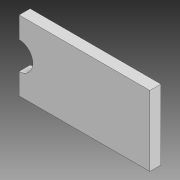
# Autodesk Inventor part: LED Backing
Saved by Autodesk Inventor 2020 (Build 240168000, 168)
## iProperties
Created: 2020-08-04
Part Number: LED Backing
Material: Generic
Document SubType Name: Modeling
Designer: DDeGo
Density: 1 g/cm^3
Appearance: Default
Author: DDeGo
Autodesk Inventor part; units mm, degrees
ref_plane "YZ Plane" through (0, 0, 0) normal (1, 0, 0) x (0, 1, 0)
ref_plane "XZ Plane" through (0, 0, 0) normal (0, 1, 0) x (-1, 0, 0)
ref_plane "XY Plane" through (0, 0, 0) normal (0, 0, 1) x (1, 0, 0)
sketch "Sketch1" plane through (0, 0, 0) normal (0, 0, 1) x (1, 0, 0)
  line L0 (-11.85, -6.35) -> (11.85, -6.35)
  line L1 (11.85, -6.35) -> (11.85, 6.35)
  line L2 (11.85, 6.35) -> (-11.85, 6.35)
  line L3 (-11.85, 6.35) -> (-11.85, 2.5)
  line L4 (-11.85, -6.35) -> (11.85, 6.35) construction
  line L5 (11.85, -6.35) -> (-11.85, 6.35) construction
  arc A0 (-11.85, -2.5) -> (-11.85, 2.5) centre (-11.85, 0) ccw
  line L6 (-11.85, 2.5) -> (-11.85, -2.5) construction
  line L7 (-11.85, -2.5) -> (-11.85, -6.35)
  line L8 (-11.85, 0) -> (0, 0) construction
  dimension "d0" = 12.7
  dimension "d1" = 23.7
  dimension "d2" = 2.5
  constraints: 18 end point, 4 parallel, 3 midpoint, 2 horizontal, 2 point on circle, 1 centre point, 1 perpendicular
  measures "d0" distance of L0.end L1.end
  measures "d1" distance of L0.start L0.end
  measures "d2" radius of A0
extrude "Extrusion1" add sketch "Sketch1" along normal blind 2
body "Solid1"
